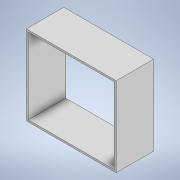
# Autodesk Inventor part: expected_size
Saved by Autodesk Inventor 2021 (Build 250183000, 183)
## iProperties
Created: 2024-04-22
Part Number: expected_size
Material: Generic
Document SubType Name: Modeling
Designer: Toby
Density: 1 g/cm^3
Appearance: Default
Author: Toby
Autodesk Inventor part; units mm, degrees
ref_plane "YZ Plane" through (0, 0, 0) normal (1, 0, 0) x (0, 1, 0)
ref_plane "XZ Plane" through (0, 0, 0) normal (0, 1, 0) x (-1, 0, 0)
ref_plane "XY Plane" through (0, 0, 0) normal (0, 0, 1) x (1, 0, 0)
sketch "Sketch1" plane through (0, 0, 0) normal (0, 0, 1) x (1, 0, 0)
  line L0 (-40.6, 40.6) -> (51.4, 40.6)
  line L1 (51.4, 40.6) -> (51.4, -40.6)
  line L2 (51.4, -40.6) -> (-40.6, -40.6)
  line L3 (-40.6, -40.6) -> (-40.6, 40.6)
  line L4 (-42.6, 42.6) -> (53.4, 42.6)
  line L5 (53.4, 42.6) -> (53.4, -42.6)
  line L6 (53.4, -42.6) -> (-42.6, -42.6)
  line L7 (-42.6, -42.6) -> (-42.6, 42.6)
  point P0 (0, 0)
  dimension "d0" = 92
  dimension "d1" = 81.2
  dimension "d2" = 40.6
  dimension "d3" = 40.6
  dimension "d4" = 2
  dimension "d5" = 2
  dimension "d6" = 2
  dimension "d7" = 2
  constraints: 16 end point, 4 parallel, 2 horizontal, 2 perpendicular
  measures "d0" distance of L0.start L0.end
  measures "d1" distance of L2.end L0.start
  measures "d2" distance from line of point (0, 0) L0
  measures "d3" distance from line of point (0, 0) L3
  measures "d4" distance between parallel lines of L0 L4
  measures "d5" distance between parallel lines of L3 L7
  measures "d6" distance between parallel lines of L6 L2
  measures "d7" distance between parallel lines of L5 L1
extrude "Extrusion1" add sketch "Sketch1" along normal blind 40
body "Solid1"
